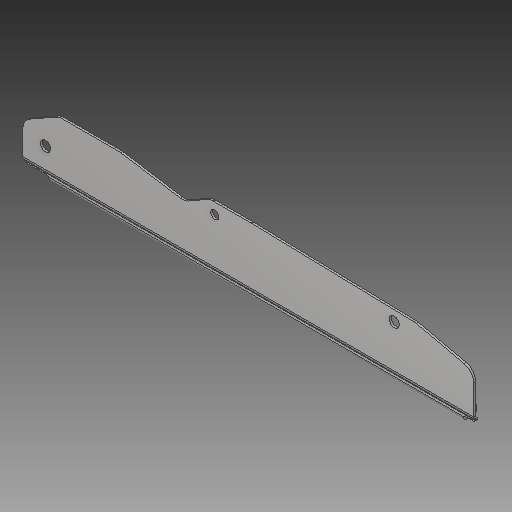
# Autodesk Inventor part: 311-01
Saved by Autodesk Inventor 2019 (Build 230136000, 136)
## iProperties
Company: Autodesk Inc.
Created: 2017-07-21
Part Number: 311-01
Material: Steel, Mild
Document SubType Name: Sheet Metal
Designer: Autodesk Inc.
Mass: 510.076 g
Surface Area: 671.482 cm^2
Volume: 64.9778 cm^3
Density: 7.85 g/cm^3
Sheet Metal Rule: Default_mm
Appearance: Anodized - Gray
Description: CHASSIS BASE
Author: Inventor
Autodesk Inventor part; units mm, degrees
ref_plane "YZ Plane" through (0, 0, 0) normal (1, 0, 0) x (0, 1, 0)
ref_plane "XZ Plane" through (0, 0, 0) normal (0, 1, 0) x (-1, 0, 0)
ref_plane "XY Plane" through (0, 0, 0) normal (0, 0, 1) x (1, 0, 0)
sketch "Sketch1" plane through (0, 0, 0) normal (0, 0, 1) x (1, 0, 0)
  line L0 (0, -50.842275) -> (0, -19.842275)
  line L1 (0, -19.842275) -> (35, 0)
  line L2 (35, 0) -> (94, 0)
  line L3 (94, 0) -> (157, -9.97822)
  line L4 (157, -9.97822) -> (181, 4)
  line L5 (181, 4) -> (221, 4)
  line L6 (221, 4) -> (380, 0.057725)
  line L7 (380, 0.057725) -> (437, -12.842275)
  line L8 (0, -50.842275) -> (437, -50.842275)
  line L9 (0, 0) -> (0, -61.810731)
  line L10 (437, -50.842275) -> (437, -12.842275)
  point P0 (0, 0)
  dimension "d0" = 50.84228
  dimension "d1" = 31
  dimension "d2" = 35
  dimension "d3" = 59
  dimension "d4" = 9
  dimension "d5" = 4
  dimension "d6" = 40
  dimension "d7" = 38
  dimension "d8" = 57
  dimension "d9" = 437
  dimension "d10" = 63
  dimension "d11" = 24
  dimension "d13" = 50.9
  measures "d0" distance from line of L9.start L8
  measures "d1" distance of L0.start L0.end
  measures "d2" distance of L9.start L1.end
  measures "d3" distance of L1.end L2.end
  measures "d4" angle of L2 L3
  measures "d5" distance between parallel lines of L5 L2
  measures "d6" distance of L4.end L5.end
  measures "d7" distance of L8.end L7.end
  measures "d8" distance from line of L6.end L10
  measures "d9" distance between parallel lines of L10 L0
  measures "d10" horizontal distance of L2.end L3.end
  measures "d11" horizontal distance of L4.end L3.end
  measures "d13" distance from line of L8 L6.end
extrude "Plate1" add sketch "Sketch1" along normal blind 2
sketch "Sketch2" plane through (0, -50.842275, 0) normal (-1, 0, 0) x (0, 0, 1)
  line L0 (-2, -4.472136) -> (-2, -6.722136)
  line L1 (-4, -8.722136) -> (-9, -8.722136)
  line L2 (-11, -6.722136) -> (-11, -1.3)
  line L3 (2, 0) -> (2, 0)
  arc A0 (-0.666667, -1.490712) -> (0, 0) centre (-2, 0) ccw
  arc A1 (-0.666667, -1.490712) -> (-2, -4.472136) centre (2, -4.472136) ccw
  arc A2 (-4, -8.722136) -> (-2, -6.722136) centre (-4, -6.722136) ccw
  arc A3 (-11, -6.722136) -> (-9, -8.722136) centre (-9, -6.722136) ccw
  line L4 (0, 0) -> (0, 31) construction
  point P0 (0, 50.842275)
  point P1 (2, 50.842279)
  dimension "d17" = 9
  dimension "d23" = 4
  dimension "d25" = 2
  dimension "d26" = 2
  dimension "d27" = 2
  dimension "d29" = 0.66667
  dimension "d30" = 2.25
  measures "d17" distance between parallel lines of L2 L0
  measures "d23" radius of A1
  measures "d25" radius of A0
  measures "d26" radius of A2
  measures "d27" radius of A3
  measures "d29" distance from line of L4 A0.start
  measures "d30" distance of L0.start L0.end
contour flange "Contour Flange1" sketch "Sketch2" thickness 2 bend radius 2 curves A0 A1 L0 A2 L1 A3 L2 edges at (218.5, -50.842275, 0) running between points at (437, -50.842275, 0) (0, -50.842275, 0)
bend "Bend1"
corner "Corner1"
sketch "Sketch3" plane through (0, -61.564411, -9) normal (-1, 0, 0) x (0, 0, 1)
  line L0 (9, 10.722136) -> (11, 10.722136)
  arc A0 (5, 2) -> (7, 4) centre (5, 4) ccw
  arc A1 (5, 0) -> (9, 4) centre (5, 4) ccw
  line L1 (0, 0) -> (5, 0)
  line L2 (0, 2) -> (5, 2)
  arc A2 (-2, 4) -> (0, 2) centre (0, 4) ccw
  arc A3 (-4, 4) -> (0, 0) centre (0, 4) ccw
  line L3 (-4, 9.422136) -> (-4, 4)
  line L4 (-2, 9.422136) -> (-2, 4)
  line L5 (-2, 9.422136) -> (-4, 9.422136)
  line L6 (7, 5.122136) -> (9, 5.122136)
  line L7 (9, 5.122136) -> (9, 4)
  line L8 (9, 4) -> (7, 4)
  line L9 (7, 4) -> (7, 5.122136)
  point P0 (9, 61.564411)
  point P1 (2, 26.833476)
  dimension "d41" = 5.6
  constraints: 8 end point, 2 parallel, 1 horizontal, 1 perpendicular
  measures "d41" distance between parallel lines of L0 L6
extrude "Extrusion1" cut sketch "Sketch3" against normal blind 23
sketch "Sketch4" plane through (437, -61.564411, -4) normal (1, 0, 0) x (0, 0, -1)
  line L0 (-4, 4) -> (-2, 4)
  line L1 (-4, 5.122136) -> (-4, 4)
  line L2 (-2, 5.122136) -> (-4, 5.122136)
  line L3 (-2, 4) -> (-2, 5.122136)
  line L4 (0, 2) -> (0, 0)
  arc A0 (-2, 4) -> (0, 2) centre (0, 4) ccw
  line L5 (-2, 4) -> (-4, 4)
  arc A1 (-4, 4) -> (0, 0) centre (0, 4) ccw
  line L6 (5, 2) -> (5, 0)
  line L7 (5, 2) -> (0, 2)
  line L8 (0, 2) -> (0, 0)
  line L9 (0, 0) -> (5, 0)
  line L10 (7, 4) -> (9, 4)
  arc A2 (5, 2) -> (7, 4) centre (5, 4) ccw
  line L11 (5, 2) -> (5, 0)
  arc A3 (5, 0) -> (9, 4) centre (5, 4) ccw
  line L12 (7, 4) -> (9, 4)
  line L13 (9, 4) -> (9, 9.422136)
  line L14 (7, 9.422136) -> (9, 9.422136)
  line L15 (7, 9.422136) -> (7, 4)
  point P0 (-4, 61.564411)
extrude "Extrusion2" cut sketch "Sketch4" against normal blind 12
fillet "Fillet1" radius 12 8 edges at (437, -12.8423, 1) (380, 0.0577, 1) (221, 4, 1) (181, 4, 1) (157, -9.9782, 1) (94, 0, 1) (35, 0, 1) (0, -19.8423, 1)
fillet "Fillet2" radius 4 2 edges at (425, -52.1423, -12) (23, -52.1423, -12)
fillet "Fillet3" radius 2 4 edges at (0, -56.4423, -1) (23, -56.4423, -1) (437, -56.4423, -1) (425, -56.4423, -1)
sketch "Sketch5" plane through (0, 0, 0) normal (0, 0, -1) x (-1, 0, 0)
  line L0 (-425, -61.564411) -> (-23, -61.564411)
  point P0 (0, 0)
  point P1 (-22, -31.064411)
  point P2 (-186, -6.564411)
  point P3 (-360, -9.564411)
  dimension "d65" = 22
  dimension "d68" = 186
  dimension "d70" = 360
  dimension "d86" = 52
  dimension "d87" = 30.5
  dimension "d88" = 55
  constraints: 1 other
  measures "d65" horizontal distance of point (-22, -31.064) point (0, 0)
  measures "d68" horizontal distance of point (0, 0) point (-186, -6.564)
  measures "d70" horizontal distance of point (-360, -9.564) point (0, 0)
  measures "d86" distance from line of point (-360, -9.564) L0
  measures "d87" distance from line of L0 point (-22, -31.064)
  measures "d88" distance from line of L0 point (-186, -6.564)
hole "Hole1" at (22, -31.064411, 0) at (360, -9.564411, 0) direction (0, 0, 1) diameter 10 end through all
hole "Hole2" at (186, -6.564411, 0) direction (0, 0, 1) diameter 8.15 end through all
equation "\"d77\" = Thickness"
equation "\"d84\" = Thickness"
equation "\"d12\" = Thickness"
equation "\"d31\" = BendReliefWidth"
equation "\"d32\" = BendReliefDepth"
equation "\"d33\" = MinimumRemnant"
equation "\"d34\" = TransitionRadius"
equation "\"d35\" = BendRadius"
equation "\"d37\" = CornerReliefSize"
equation "\"d38\" = GapSize"
equation "\"d39\" = JacobiRadiusSize"
equation "\"BendRadius\" = Thickness"
equation "\"BendReliefWidth\" = Thickness"
equation "\"BendReliefDepth\" = 0.5 * Thickness"
equation "\"CornerReliefSize\" = 4 * Thickness"
equation "\"MinimumRemnant\" = 2 * Thickness"
equation "\"TransitionRadius\" = BendRadius"
equation "\"JacobiRadiusSize\" = BendRadius"
equation "\"GapSize\" = Thickness"
equation "\"Thickness\" = 2"
body "Solid1"
